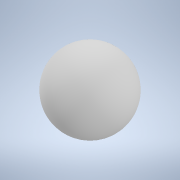
# Autodesk Inventor part: sphere
Saved by Autodesk Inventor 2021 (Build 250183000, 183)
## iProperties
Created: 2020-05-07
Part Number: sphere
Material: Generic
Document SubType Name: Modeling
Designer: david
Density: 1 g/cm^3
Appearance: Default
Author: david
Autodesk Inventor part; units mm, degrees
ref_plane "YZ Plane" through (0, 0, 0) normal (1, 0, 0) x (0, 1, 0)
ref_plane "XZ Plane" through (0, 0, 0) normal (0, 1, 0) x (-1, 0, 0)
ref_plane "XY Plane" through (0, 0, 0) normal (0, 0, 1) x (1, 0, 0)
sketch "Sketch1" plane through (0, 0, 0) normal (0, 1, 0) x (-1, 0, 0)
  arc A0 (2.2081, -15.5253) -> (22.1261, -15.5253) centre (12.1671, -15.5253) ccw
  line L0 (22.1261, -15.5253) -> (2.2081, -15.5253)
  point P0 (0, 0)
  dimension "d0" = 90
  constraints: 2 end point, 2 point on circle, 1 centre point, 1 horizontal
revolve "Revolution1" add sketch "Sketch1" angle 360 about axis through (-22.1261, 0, -15.5253) along (1, 0, 0)
body "Solid1"
